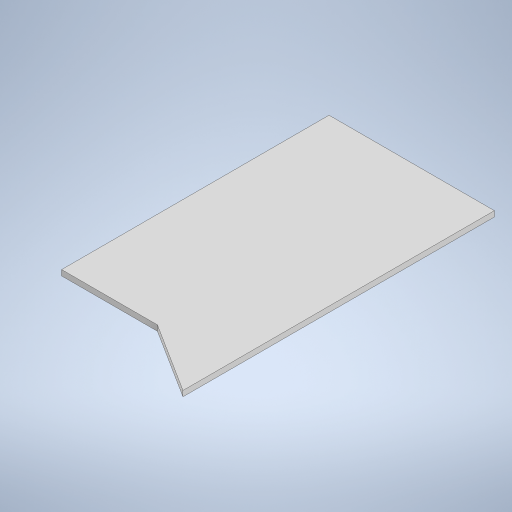
# Autodesk Inventor part: tapa4
Saved by Autodesk Inventor 2024 (Build 280153000, 153)
## iProperties
Created: 2024-05-27
Part Number: tapa4
Material: Generic
Document SubType Name: Modeling
Designer: samue
Density: 1 g/cm^3
Appearance: Default
Author: samue
Autodesk Inventor part; units mm, degrees
ref_plane "YZ Plane" through (0, 0, 0) normal (1, 0, 0) x (0, 1, 0)
ref_plane "XZ Plane" through (0, 0, 0) normal (0, 1, 0) x (-1, 0, 0)
ref_plane "XY Plane" through (0, 0, 0) normal (0, 0, 1) x (1, 0, 0)
sketch "Sketch1" plane through (0, 0, 0) normal (0, 1, 0) x (-1, 0, 0)
  line L0 (0, 11.5371) -> (0, -101.4629)
  line L1 (0, -101.4629) -> (60, -101.4629)
  line L2 (0, 11.5371) -> (25.2319, -4.4338)
  line L3 (25.2319, -4.4338) -> (60, -4.4338)
  line L4 (60, -4.4338) -> (60, -101.4629)
  point P0 (0, 0)
  dimension "d0" = 113
  dimension "d2" = 60
  constraints: 10 end point, 2 perpendicular, 1 horizontal, 1 vertical
  measures "d0" distance of L0.start L0.end
  measures "d2" distance of L0.end L1.end
extrude "Extrusion1" add sketch "Sketch1" along normal blind 2
body "Solid1"
